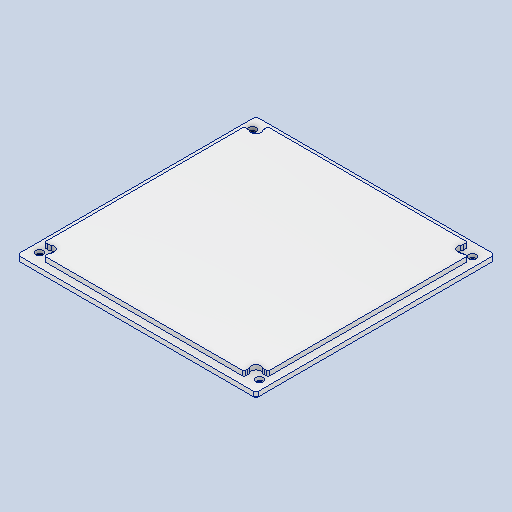
# Autodesk Inventor part: TopPanel
Saved by Autodesk Inventor 2023 (Build 270158000, 158)
## iProperties
Created: 2022-08-01
Part Number: TopPanel
Material: Aluminum 6061
Document SubType Name: Modeling
Designer: Aditya Bansal
Density: 2.7 g/cm^3
Appearance: Aluminum - Flat
Author: Aditya Bansal
Autodesk Inventor part; units mm, degrees
ref_plane "YZ Plane" through (0, 0, 0) normal (1, 0, 0) x (0, 1, 0)
ref_plane "XZ Plane" through (0, 0, 0) normal (0, 1, 0) x (-1, 0, 0)
ref_plane "XY Plane" through (0, 0, 0) normal (0, 0, 1) x (1, 0, 0)
sketch "Sketch1" plane through (0, 0, 0) normal (0, 1, 0) x (-1, 0, 0)
  line L0 (0, 0) -> (100, 0)
  line L1 (100, 0) -> (100, -100)
  line L2 (100, -100) -> (0, -100)
  line L3 (0, -100) -> (0, 0)
  dimension "d0" = 100
  constraints: 8 end point, 2 parallel, 2 perpendicular, 1 horizontal
  measures "d0" distance of L0.end L1.end
extrude "Extrusion1" add sketch "Sketch1" along normal blind 3
sketch "Sketch2" plane through (0, 3, 0) normal (0, 1, 0) x (1, 0, 0)
  line L0 (0, 100) -> (-100, 100) construction
  line L1 (0, 0) -> (0, 100) construction
  line L2 (-100, 100) -> (0, 100) construction
  line L3 (0, 100) -> (0, 97) construction
  line L4 (0, 97) -> (-100, 97) construction
  line L5 (-100, 97) -> (-100, 100) construction
  line L6 (-100, 0) -> (0, 0) construction
  line L7 (0, 0) -> (-100, 0) construction
  line L8 (-100, 0) -> (-100, 3) construction
  line L9 (-100, 3) -> (0, 3) construction
  line L10 (0, 3) -> (0, 0) construction
  line L11 (-100, 97) -> (-97, 97) construction
  line L12 (-97, 92) -> (-97, 8) construction
  line L13 (-97.6517, 3) -> (-100, 3) construction
  line L14 (-100, 3) -> (-100, 97) construction
  line L15 (-97.6517, 3) -> (-92, 3) construction
  line L16 (-92, 3) -> (-92, 8) construction
  line L17 (-92, 8) -> (-97, 8) construction
  line L18 (-97.6517, 3.25) -> (-97.6517, 3) construction
  line L19 (-97, 97) -> (-92, 97) construction
  line L20 (-92, 97) -> (-92, 92) construction
  line L21 (-92, 92) -> (-97, 92) construction
  line L22 (-97, 96.75) -> (-97, 97) construction
  line L23 (0, 97) -> (-3.4863, 97) construction
  line L24 (-3, 92) -> (-3, 8) construction
  line L25 (-2.3483, 3) -> (0, 3) construction
  line L26 (0, 3) -> (0, 97) construction
  line L27 (-2.3483, 3) -> (-8, 3) construction
  line L28 (-8, 3) -> (-8, 8) construction
  line L29 (-8, 8) -> (-3, 8) construction
  line L30 (-2.3483, 3.25) -> (-2.3483, 3) construction
  line L31 (-3.4863, 97) -> (-8, 97) construction
  line L32 (-8, 97) -> (-8, 92) construction
  line L33 (-8, 92) -> (-3, 92) construction
  line L34 (-3.4863, 96.75) -> (-3.4863, 97) construction
  line L35 (-96.75, 91.75) -> (-96.75, 8.25)
  line L36 (-96.75, 8.25) -> (-91.75, 8.25)
  line L37 (-91.75, 8.25) -> (-91.75, 3.25)
  line L38 (-91.75, 3.25) -> (-8.25, 3.25)
  line L39 (-8.25, 3.25) -> (-8.25, 8.25)
  line L40 (-8.25, 8.25) -> (-3.25, 8.25)
  line L41 (-3.25, 8.25) -> (-3.25, 91.75)
  line L42 (-3.25, 91.75) -> (-8.25, 91.75)
  line L43 (-8.25, 91.75) -> (-8.25, 96.75)
  line L44 (-8.25, 96.75) -> (-91.75, 96.75)
  line L45 (-91.75, 96.75) -> (-91.75, 91.75)
  line L46 (-91.75, 91.75) -> (-96.75, 91.75)
  arc A0 (-91.75, 5.4216) -> (-94.5784, 8.25) centre (-93.1642, 6.8358) ccw
  line L47 (-91.75, 8.25) -> (-93.1642, 6.8358) construction
  arc A1 (-5.4216, 8.25) -> (-8.25, 5.4216) centre (-6.8358, 6.8358) ccw
  line L48 (-8.25, 8.25) -> (-6.8358, 6.8358) construction
  line L49 (-96.75, 50) -> (-3.25, 50) construction
  line L50 (-50, 96.75) -> (-50, 3.25) construction
  arc A2 (-94.5784, 91.75) -> (-91.75, 94.5784) centre (-93.1642, 93.1642) ccw
  arc A3 (-8.25, 94.5784) -> (-5.4216, 91.75) centre (-6.8358, 93.1642) ccw
  point P0 (-5.4216, 91.75)
  point P1 (-8.25, 94.5784)
  point P2 (-91.75, 94.5784)
  dimension "d4" = 100
  dimension "d5" = 5
  dimension "d6" = 5
  dimension "d7" = 3
  dimension "d8" = 0.25
  dimension "d9" = 0.25
  dimension "d10" = 0.25
  dimension "d11" = 0.25
  dimension "d12" = 0.25
  dimension "d13" = 0.25
  dimension "d14" = 0.25
  dimension "d15" = 0.25
  dimension "d16" = 2
  dimension "d22" = 3
  dimension "d23" = 3
  constraints: 96 end point, 19 point on line, 18 parallel, 17 perpendicular, 10 point on circle, 8 collinear, 8 horizontal, 6 symmetric about line, 4 centre point, 4 midpoint, 1 equal radius, 2 other
  measures "d4" distance of L1.start L0.start
  measures "d5" distance of L12.start L20.end
  measures "d6" distance of L19.end L20.end
  measures "d7" distance between parallel lines of L14 L12
  measures "d8" distance between parallel lines of L38 L9
  measures "d9" distance between parallel lines of L4 L44
  measures "d10" distance between parallel lines of L24 L41
  measures "d11" distance between parallel lines of L12 L35
  measures "d12" distance between parallel lines of L17 L36
  measures "d13" distance between parallel lines of L16 L37
  measures "d14" distance between parallel lines of L39 L28
  measures "d15" distance between parallel lines of L21 L46
  measures "d16" radius of A0
  measures "d22" distance between parallel lines of L26 L24
  measures "d23" distance between parallel lines of L6 L9
extrude "Extrusion2" add sketch "Sketch2" along normal blind 2 contours L46 A2 L45 L44 L43 A3 L42 L41 L40 A1 L39 L38 L37 A0 L36 L35
fillet "Fillet1" radius 2 8 edges at (-91.75, 4, -94.5784) (-94.5784, 4, -91.75) (-94.5784, 4, -8.25) (-91.75, 4, -5.4216) (-8.25, 4, -5.4216) (-5.4216, 4, -8.25) (-8.25, 4, -94.5784) (-5.4216, 4, -91.75)
fillet "Fillet2" radius 0.5 8 edges at (-96.75, 4, -8.25) (-91.75, 4, -3.25) (-8.25, 4, -3.25) (-3.25, 4, -8.25) (-3.25, 4, -91.75) (-8.25, 4, -96.75) (-91.75, 4, -96.75) (-96.75, 4, -91.75)
sketch "Sketch4" plane through (0, 0, 0) normal (0, -1, 0) x (1, 0, 0)
  line L0 (0, -100) -> (-100, -100) construction
  line L1 (0, -100) -> (-100, -100) construction
  line L2 (-100, -100) -> (-100, -97) construction
  line L3 (-100, -97) -> (0, -97) construction
  line L4 (0, -97) -> (0, -100) construction
  line L5 (-100, -100) -> (-100, 0) construction
  line L6 (0, 0) -> (0, -100) construction
  line L7 (-100, 0) -> (0, 0) construction
  line L8 (0, 0) -> (0, -3) construction
  line L9 (0, -3) -> (-100, -3) construction
  line L10 (-100, -3) -> (-100, 0) construction
  line L11 (0, -97) -> (-8.25, -97) construction
  line L12 (-8.25, -97) -> (-8.25, -91.75) construction
  line L13 (-8.25, -91.75) -> (0, -91.75) construction
  line L14 (0, -91.75) -> (0, -97) construction
  line L15 (-100, -97) -> (-91.75, -97) construction
  line L16 (-91.75, -97) -> (-91.75, -91.75) construction
  line L17 (-91.75, -91.75) -> (-100, -91.75) construction
  line L18 (-100, -91.75) -> (-100, -97) construction
  line L19 (0, -3) -> (-8.25, -3) construction
  line L20 (-8.25, -3) -> (-8.25, -8.25) construction
  line L21 (-8.25, -8.25) -> (0, -8.25) construction
  line L22 (0, -8.25) -> (0, -3) construction
  line L23 (-100, -3) -> (-91.75, -3) construction
  line L24 (-91.75, -3) -> (-91.75, -8.25) construction
  line L25 (-91.75, -8.25) -> (-100, -8.25) construction
  line L26 (-100, -8.25) -> (-100, -3) construction
  arc A0 (-96.75, -91.25) -> (-96.25, -91.75) centre (-96.25, -91.25) ccw construction
  line L27 (-96.75, -91.25) -> (-96.75, -8.75) construction
  arc A1 (-96.25, -8.25) -> (-96.75, -8.75) centre (-96.25, -8.75) ccw construction
  line L28 (-96.25, -8.25) -> (-95.2482, -8.25) construction
  arc A2 (-94.2062, -8.5429) -> (-95.2482, -8.25) centre (-95.2482, -10.25) ccw construction
  arc A3 (-94.2062, -8.5429) -> (-91.4571, -5.7938) centre (-93.1642, -6.8358) ccw construction
  arc A4 (-91.75, -4.7518) -> (-91.4571, -5.7938) centre (-89.75, -4.7518) ccw construction
  line L29 (-91.75, -4.7518) -> (-91.75, -3.75) construction
  arc A5 (-91.25, -3.25) -> (-91.75, -3.75) centre (-91.25, -3.75) ccw construction
  line L30 (-91.25, -3.25) -> (-8.75, -3.25) construction
  arc A6 (-8.25, -3.75) -> (-8.75, -3.25) centre (-8.75, -3.75) ccw construction
  line L31 (-8.25, -3.75) -> (-8.25, -4.7518) construction
  arc A7 (-8.5429, -5.7938) -> (-8.25, -4.7518) centre (-10.25, -4.7518) ccw construction
  arc A8 (-8.5429, -5.7938) -> (-5.7938, -8.5429) centre (-6.8358, -6.8358) ccw construction
  arc A9 (-4.7518, -8.25) -> (-5.7938, -8.5429) centre (-4.7518, -10.25) ccw construction
  line L32 (-4.7518, -8.25) -> (-3.75, -8.25) construction
  arc A10 (-3.25, -8.75) -> (-3.75, -8.25) centre (-3.75, -8.75) ccw construction
  line L33 (-3.25, -8.75) -> (-3.25, -91.25) construction
  arc A11 (-3.75, -91.75) -> (-3.25, -91.25) centre (-3.75, -91.25) ccw construction
  line L34 (-3.75, -91.75) -> (-4.7518, -91.75) construction
  arc A12 (-5.7938, -91.4571) -> (-4.7518, -91.75) centre (-4.7518, -89.75) ccw construction
  arc A13 (-5.7938, -91.4571) -> (-8.5429, -94.2062) centre (-6.8358, -93.1642) ccw construction
  arc A14 (-8.25, -95.2482) -> (-8.5429, -94.2062) centre (-10.25, -95.2482) ccw construction
  line L35 (-8.25, -95.2482) -> (-8.25, -96.25) construction
  arc A15 (-8.75, -96.75) -> (-8.25, -96.25) centre (-8.75, -96.25) ccw construction
  line L36 (-8.75, -96.75) -> (-91.25, -96.75) construction
  arc A16 (-91.75, -96.25) -> (-91.25, -96.75) centre (-91.25, -96.25) ccw construction
  line L37 (-91.75, -96.25) -> (-91.75, -95.2482) construction
  arc A17 (-91.4571, -94.2062) -> (-91.75, -95.2482) centre (-89.75, -95.2482) ccw construction
  arc A18 (-91.4571, -94.2062) -> (-94.2062, -91.4571) centre (-93.1642, -93.1642) ccw construction
  arc A19 (-95.2482, -91.75) -> (-94.2062, -91.4571) centre (-95.2482, -89.75) ccw construction
  line L38 (-95.2482, -91.75) -> (-96.25, -91.75) construction
  line L39 (0, -100) -> (-100, -100) construction
  line L40 (0, 0) -> (0, -100) construction
  line L41 (-100, 0) -> (0, 0) construction
  line L42 (-100, -100) -> (-100, 0) construction
  point P0 (-4, -5.5)
  point P1 (-4, -94.5)
  point P2 (-96, -94.5)
  point P3 (-96, -5.5)
  dimension "d50" = 3
  dimension "d51" = 8.25
  dimension "d52" = 4
  dimension "d53" = 5.25
  dimension "d54" = 2.5
  dimension "d55" = 4
  dimension "d56" = 2.5
  constraints: 48 end point, 13 parallel, 8 collinear, 6 horizontal, 6 perpendicular, 2 horizontal alignment, 2 vertical alignment, 1 point on line
  measures "d50" distance between parallel lines of L0 L3
  measures "d51" distance of L20.end L21.end
  measures "d52" distance from line of point (-4, -5.5) L22
  measures "d53" distance of L19.end L20.end
  measures "d54" distance from line of point (-4, -5.5) L9
  measures "d55" distance from line of L5 point (-96, -5.5)
  measures "d56" distance from line of L11 point (-4, -94.5)
hole "Hole1" at (-4, 0, -5.5) at (-4, 0, -94.5) at (-96, 0, -94.5) at (-96, 0, -5.5) direction (0, 1, 0) diameter 3.2 end through all countersink diameter 6.3 countersink angle 90 clearance for "Flat Head Machine Screw" size "M3" standard "Ansi Metric M Profile"
chamfer "Chamfer1" distance 1 angle 45 8 edges at (-50, 0, -100) (0, 0, -50) (-50, 0, 0) (-100, 0, -50) (0, 1.5, 0) (-100, 1.5, 0) (-100, 1.5, -100) (0, 1.5, -100)
equation "\"d6\" = d5"
equation "\"d9\" = d8"
equation "\"d10\" = d9"
equation "\"d11\" = d9"
equation "\"d12\" = d11"
equation "\"d13\" = d12"
equation "\"d14\" = d13"
equation "\"d15\" = d12"
equation "\"d23\" = d22"
body "Solid1"
